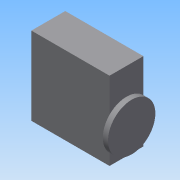
# Autodesk Inventor part: moteur euger 16_03
Saved by Autodesk Inventor 2013 (Build 170138000, 138)
## iProperties
Created: 2012-11-14
Part Number: moteur euger 16_03
Material: Générique
Document SubType Name: Modeling
Designer: Aegir
Density: 1 g/cm^3
Author: Aegir
Autodesk Inventor part; units mm, degrees
ref_plane "YZ Plane" through (0, 0, 0) normal (1, 0, 0) x (0, 1, 0)
ref_plane "XZ Plane" through (0, 0, 0) normal (0, 1, 0) x (-1, 0, 0)
ref_plane "XY Plane" through (0, 0, 0) normal (0, 0, 1) x (1, 0, 0)
sketch "Esquisse1" plane through (0, 0, 0) normal (0, 1, 0) x (-1, 0, 0)
  line L0 (0, 0) -> (-30, 0)
  line L1 (-30, 0) -> (-30, 30)
  line L2 (-30, 30) -> (0, 30)
  line L3 (0, 30) -> (0, 0)
  dimension "d0" = 30
  dimension "d2" = 30
  constraints: 8 end point, 2 parallel, 1 horizontal, 1 perpendicular
  measures "d0" distance of L1.end L2.end
  measures "d2" distance of L0.end L1.end
extrude "Extrusion1" add sketch "Esquisse1" along normal blind 13
sketch "Esquisse2" plane through (30, 0, 30) normal (1, 0, 0) x (0, 0, -1)
  circle A0 centre (19.3193, 6.5) radius 9.0917
  constraints: 1 centre point
extrude "Extrusion2" add sketch "Esquisse2" along normal blind 2
